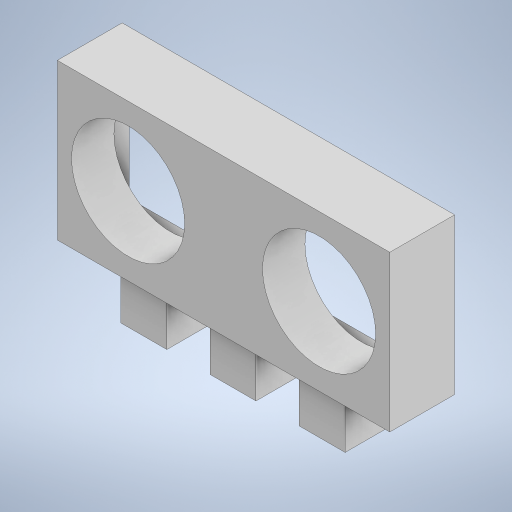
# Autodesk Inventor part: Sonar
Saved by Autodesk Inventor 2024.1 (Build 281209000, 209)
## iProperties
Created: 2024-05-13
Part Number: Sonar
Material: Generic
Document SubType Name: Modeling
Designer: cyan924
Density: 1 g/cm^3
Appearance: Default
Author: cyan924
Autodesk Inventor part; units mm, degrees
ref_plane "YZ Plane" through (0, 0, 0) normal (1, 0, 0) x (0, 1, 0)
ref_plane "XZ Plane" through (0, 0, 0) normal (0, 1, 0) x (-1, 0, 0)
ref_plane "XY Plane" through (0, 0, 0) normal (0, 0, 1) x (1, 0, 0)
sketch "Sketch1" plane through (0, 0, 0) normal (0, 0, 1) x (1, 0, 0)
  line L0 (0, 0) -> (45, 0) construction
  line L1 (45, 0) -> (45, 20) construction
  line L2 (45, 20) -> (0, 20) construction
  line L3 (0, 20) -> (0, 0) construction
  line L4 (0, 0) -> (9, 0) construction
  line L5 (9, 0) -> (9, 10) construction
  line L6 (45, 0) -> (36, 0) construction
  line L7 (36, 0) -> (36, 10) construction
  circle A0 centre (36, 10) radius 8
  circle A1 centre (9, 10) radius 8
  line L8 (45, 0) -> (46, 0) construction
  line L9 (46, 0) -> (46, -1) construction
  line L10 (0, 20) -> (-1, 20) construction
  line L11 (-1, 20) -> (-1, 21) construction
  line L12 (-1, 21) -> (46, 21)
  line L13 (46, 21) -> (46, -1)
  line L14 (46, -1) -> (-1, -1)
  line L15 (-1, -1) -> (-1, 21)
  line L16 (45, 0) -> (0, 0)
  line L17 (0, 0) -> (0, 20)
  line L18 (0, 20) -> (45, 20)
  line L19 (45, 20) -> (45, 0)
  dimension "d2" = 45
  dimension "d3" = 20
  dimension "d4" = 9
  dimension "d5" = 10
  dimension "d6" = 9
  dimension "d7" = 10
  dimension "d8" = 16
  dimension "d9" = 16
  dimension "d10" = 1
  dimension "d11" = 1
  dimension "d12" = 1
  dimension "d13" = 1
  constraints: 40 end point, 7 perpendicular, 6 parallel, 5 horizontal, 2 centre point, 2 coincident, 2 point on line
  measures "d2" distance of L2.end L1.end
  measures "d3" distance of L1.end L0.end
  measures "d4" distance of L0.start L4.end
  measures "d5" distance of L4.end L5.end
  measures "d6" distance of L0.end L6.end
  measures "d7" distance of L6.end L7.end
  measures "d8" diameter of A0
  measures "d9" diameter of A1
  measures "d10" distance of L0.end L8.end
  measures "d11" distance of L8.end L9.end
  measures "d12" distance of L2.end L10.end
  measures "d13" distance of L10.end L11.end
extrude "Extrusion1" add sketch "Sketch1" along normal blind 9.169 contours L12 L13 L14 L15 | L16 L17 L18 L19
sketch "Sketch2" plane through (0, 0, 0) normal (0, 0, -1) x (-1, 0, 0)
  line L0 (0, 0) -> (-45, 0)
  line L1 (-45, 0) -> (-45, 20)
  line L2 (-45, 20) -> (0, 20)
  line L3 (0, 20) -> (0, 0)
  dimension "d14" = 45
  dimension "d15" = 20
  constraints: 8 end point, 2 parallel, 1 horizontal, 1 perpendicular
  measures "d14" distance of L1.end L2.end
  measures "d15" distance of L0.end L1.end
extrude "Extrusion2" cut sketch "Sketch2" against normal blind 3.169
sketch "Sketch3" plane through (-1, -1, 0) normal (0, -1, 0) x (1, 0, 0)
  line L0 (47, 0) -> (47, 9.169) construction
  line L1 (47, 4.5845) -> (0, 4.5845) construction
  line L2 (0, 0) -> (0, 9.169) construction
  line L3 (47, 0) -> (0, 0) construction
  line L4 (23.5, 0) -> (23.5, 9.169) construction
  line L5 (0, 9.169) -> (47, 9.169) construction
  line L6 (23.5, 4.5845) -> (23.5, 2.3345) construction
  line L7 (23.5, 2.3345) -> (21.25, 2.3345) construction
  line L8 (21.25, 2.3345) -> (13.15, 2.3345) construction
  line L9 (13.15, 2.3345) -> (8.65, 2.3345) construction
  line L10 (8.65, 2.3345) -> (0.55, 2.3345) construction
  line L11 (0.55, 2.3345) -> (-3.95, 2.3345) construction
  line L12 (-3.95, 2.3345) -> (-12.05, 2.3345) construction
  line L13 (23.5, 2.3345) -> (25.75, 2.3345) construction
  line L14 (25.75, 2.3345) -> (33.85, 2.3345) construction
  line L15 (33.85, 2.3345) -> (38.35, 2.3345) construction
  line L16 (38.35, 2.3345) -> (46.45, 2.3345) construction
  line L17 (46.45, 2.3345) -> (50.95, 2.3345) construction
  line L18 (50.95, 2.3345) -> (59.05, 2.3345) construction
  line L19 (21.25, 2.3345) -> (25.75, 2.3345)
  line L20 (25.75, 2.3345) -> (25.75, 6.8345)
  line L21 (25.75, 6.8345) -> (21.25, 6.8345)
  line L22 (21.25, 6.8345) -> (21.25, 2.3345)
  line L23 (8.65, 2.3345) -> (13.15, 2.3345)
  line L24 (13.15, 2.3345) -> (13.15, 6.8345)
  line L25 (13.15, 6.8345) -> (8.65, 6.8345)
  line L26 (8.65, 6.8345) -> (8.65, 2.3345)
  line L27 (38.35, 2.3345) -> (33.85, 2.3345)
  line L28 (33.85, 2.3345) -> (33.85, 6.8345)
  line L29 (33.85, 6.8345) -> (38.35, 6.8345)
  line L30 (38.35, 6.8345) -> (38.35, 2.3345)
  line L31 (13.15, 2.3345) -> (14.15, 2.3345) construction
  line L32 (14.15, 2.3345) -> (14.15, 1.3345) construction
  line L33 (8.65, 6.8345) -> (8.65, 7.8345) construction
  line L34 (8.65, 7.8345) -> (7.65, 7.8345) construction
  line L35 (7.65, 7.8345) -> (14.15, 7.8345)
  line L36 (14.15, 7.8345) -> (14.15, 1.3345)
  line L37 (14.15, 1.3345) -> (7.65, 1.3345)
  line L38 (7.65, 1.3345) -> (7.65, 7.8345)
  line L39 (25.75, 2.3345) -> (26.75, 2.3345) construction
  line L40 (26.75, 2.3345) -> (26.75, 1.3345) construction
  line L41 (21.25, 6.8345) -> (21.25, 7.8345) construction
  line L42 (21.25, 7.8345) -> (20.25, 7.8345) construction
  line L43 (33.85, 6.8345) -> (32.85, 6.8345) construction
  line L44 (32.85, 6.8345) -> (32.85, 7.8345) construction
  line L45 (38.35, 2.3345) -> (39.35, 2.3345) construction
  line L46 (39.35, 2.3345) -> (39.35, 1.3345) construction
  line L47 (26.75, 1.3345) -> (20.25, 1.3345)
  line L48 (20.25, 1.3345) -> (20.25, 7.8345)
  line L49 (20.25, 7.8345) -> (26.75, 7.8345)
  line L50 (26.75, 7.8345) -> (26.75, 1.3345)
  line L51 (39.35, 1.3345) -> (32.85, 1.3345)
  line L52 (32.85, 1.3345) -> (32.85, 7.8345)
  line L53 (32.85, 7.8345) -> (39.35, 7.8345)
  line L54 (39.35, 7.8345) -> (39.35, 1.3345)
  point P0 (1, 0)
  dimension "d18" = 2.25
  dimension "d19" = 2.25
  dimension "d20" = 8.1
  dimension "d21" = 4.5
  dimension "d22" = 8.1
  dimension "d23" = 4.5
  dimension "d24" = 8.1
  dimension "d25" = 2.25
  dimension "d26" = 8.1
  dimension "d27" = 4.5
  dimension "d28" = 8.1
  dimension "d29" = 4.5
  dimension "d30" = 8.1
  dimension "d31" = 4.5
  dimension "d32" = 4.5
  dimension "d33" = 4.5
  dimension "d34" = 4.5
  dimension "d35" = 4.5
  dimension "d36" = 4.5
  dimension "d37" = 1
  dimension "d38" = 1
  dimension "d39" = 1
  dimension "d40" = 1
  dimension "d41" = 1
  dimension "d42" = 1
  dimension "d43" = 1
  dimension "d44" = 1
  dimension "d45" = 1
  dimension "d46" = 1
  dimension "d47" = 1
  dimension "d48" = 1
  constraints: 102 end point, 14 point on line, 13 perpendicular, 12 parallel, 8 horizontal, 5 midpoint, 2 vertical
  measures "d18" distance of L6.start L6.end
  measures "d19" distance of L6.end L7.end
  measures "d20" distance of L7.end L8.end
  measures "d21" distance of L8.end L9.end
  measures "d22" distance of L9.end L10.end
  measures "d23" distance of L10.end L11.end
  measures "d24" distance of L11.end L12.end
  measures "d25" distance of L6.end L13.end
  measures "d26" distance of L13.end L14.end
  measures "d27" distance of L14.end L15.end
  measures "d28" distance of L15.end L16.end
  measures "d29" distance of L16.end L17.end
  measures "d30" distance of L17.end L18.end
  measures "d31" distance of L21.end L20.end
  measures "d32" distance of L20.end L19.end
  measures "d33" distance of L25.end L24.end
  measures "d34" distance of L24.end L23.end
  measures "d35" distance of L28.end L29.end
  measures "d36" distance of L27.end L28.end
  measures "d37" distance of L23.end L31.end
  measures "d38" distance of L31.end L32.end
  measures "d39" distance of L25.end L33.end
  measures "d40" distance of L33.end L34.end
  measures "d41" distance of L19.end L39.end
  measures "d42" distance of L39.end L40.end
  measures "d43" distance of L21.end L41.end
  measures "d44" distance of L41.end L42.end
  measures "d45" distance of L28.end L43.end
  measures "d46" distance of L43.end L44.end
  measures "d47" distance of L15.end L45.end
  measures "d48" distance of L45.end L46.end
extrude "Extrusion3" add sketch "Sketch3" along normal blind 7
equation "\"d2\" = wsonar"
equation "\"d3\" = hsonar"
equation "\"d10\" = thickness"
equation "\"d11\" = thickness"
equation "\"d12\" = thickness"
equation "\"d13\" = thickness"
equation "\"d14\" = wsonar"
equation "\"d15\" = hsonar"
equation "\"d18\" = 0.5 * box"
equation "\"d19\" = 0.5 * box"
equation "\"d20\" = gap"
equation "\"d21\" = box"
equation "\"d22\" = gap"
equation "\"d23\" = box"
equation "\"d24\" = gap"
equation "\"d25\" = 0.5 * box"
equation "\"d26\" = gap"
equation "\"d27\" = box"
equation "\"d28\" = gap"
equation "\"d29\" = box"
equation "\"d30\" = gap"
equation "\"d31\" = box"
equation "\"d32\" = box"
equation "\"d33\" = box"
equation "\"d34\" = box"
equation "\"d35\" = box"
equation "\"d36\" = box"
equation "\"d37\" = thickness"
equation "\"d38\" = thickness"
equation "\"d39\" = thickness"
equation "\"d40\" = thickness"
equation "\"d41\" = thickness"
equation "\"d42\" = thickness"
equation "\"d43\" = thickness"
equation "\"d44\" = thickness"
equation "\"d45\" = thickness"
equation "\"d46\" = thickness"
equation "\"d47\" = thickness"
equation "\"d48\" = thickness"
equation "\"wsonar\" = 45"
equation "\"hsonar\" = 20"
equation "\"thickness\" = 1"
equation "\"gap\" = 8.1"
equation "\"box\" = 4.5"
body "Solid1"
